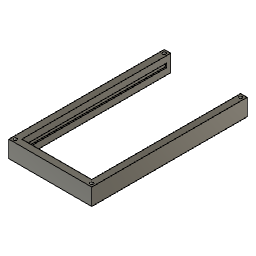
STM Holder v1 (Autodesk Fusion 360 design; units mm, degrees)
Autodesk Fusion 360 part; units mm, degrees
sketch "Sketch1" plane through (0, 0, 0) normal (0, 0, 1) x (1, 0, 0)
  line L0 (16.12, 50) -> (16.12, -69.76)
  line L1 (16.12, -69.76) -> (80, -69.76)
  line L2 (80, -69.76) -> (80, 50)
  line L3 (80, 50) -> (75, 50)
  line L4 (75, 50) -> (75, -64.76)
  line L5 (75, -64.76) -> (21.12, -64.76)
  line L6 (21.12, -64.76) -> (21.12, 50)
  line L7 (21.12, 50) -> (16.12, 50)
  circle A0 centre (18.62, 47.5) radius 1.25
  circle A1 centre (77.5, 47.5) radius 1.25
  circle A2 centre (18.62, -67.26) radius 1.25
  circle A3 centre (77.5, -67.26) radius 1.25
  dimension "d9" = 5
  dimension "d10" = 5
  dimension "d11" = 5
  dimension "d12" = 119.76
  dimension "d13" = 63.88
  dimension "d16" = 2.5
  dimension "d17" = 2.5
  dimension "d18" = 2.5
  dimension "d19" = 2.5
  dimension "d20" = 2.5
  dimension "d21" = 2.5
  dimension "d22" = 2.5
  dimension "d23" = 2.5
  dimension "d24" = 2.5
  dimension "d25" = 2.5
  dimension "d26" = 2.5
  dimension "d27" = 2.5
  dimension "d39" = 114.76
  constraint vertical L0
  constraint perpendicular L0 L1
  constraint perpendicular L1 L2
  constraint perpendicular L2 L3
  constraint perpendicular L3 L4
  constraint perpendicular L4 L5
  constraint perpendicular L5 L6
  constraint perpendicular L0 L7
  measures "d9" distance of L0.start L6.end
  measures "d10" distance of L2.end L3.end
  measures "d11" distance of L1 L4.end
  measures "d12" distance of L0.start L0.end
  measures "d13" distance of L0.end L1.end
  measures "d16" diameter of A0
  measures "d17" diameter of A1
  measures "d18" diameter of A2
  measures "d19" diameter of A3
  measures "d20" distance of L1 A2.centre
  measures "d21" distance of L0 A2.centre
  measures "d22" distance of L2 A3.centre
  measures "d23" distance of L1 A3.centre
  measures "d24" distance of L3 A1.centre
  measures "d25" distance of L2 A1.centre
  measures "d26" distance of L7 A0.centre
  measures "d27" distance of L0 A0.centre
  measures "d39" distance of L3.end L4.end
extrude "Extrude2" add sketch "Sketch1" along normal blind 18
sketch "Sketch3" plane through (0, 50, 0) normal (0, 1, 0) x (-1, 0, 0)
  line L0 (-80, 0) -> (-75, 0)
  line L1 (-75, 0) -> (-75, 18)
  line L2 (-75, 18) -> (-80, 18)
  line L3 (-80, 18) -> (-80, 0)
  line L4 (-75, 10) -> (-76, 10)
  line L5 (-76, 10) -> (-76, 13)
  line L6 (-76, 13) -> (-75, 13)
  line L7 (-75, 13) -> (-75, 10)
  dimension "d34" = 3
  dimension "d35" = 1
  dimension "d36" = 5
  constraint horizontal L4
  constraint vertical L5
  constraint horizontal L6
  constraint vertical L7
  constraint coincident L1 L4.start
  measures "d34" distance of L4.start L6.end
  measures "d35" distance of L4.start L4.end
  measures "d36" distance of L1.end L6.end
extrude "Extrude3" cut sketch "Sketch3" against normal blind 115.76 contours L1 L4 L5 L6 L7
sketch "Sketch4" plane through (0, -64.76, 0) normal (0, 1, 0) x (-1, 0, 0)
  line L0 (-75, 0) -> (-21.12, 0)
  line L1 (-21.12, 0) -> (-21.12, 18)
  line L2 (-21.12, 18) -> (-75, 18)
  line L3 (-75, 18) -> (-75, 13)
  line L4 (-75, 13) -> (-75, 10)
  line L5 (-75, 10) -> (-75, 0)
  line L6 (-75, 13) -> (-21.12, 13)
  line L7 (-21.12, 13) -> (-21.12, 9)
  line L8 (-21.12, 9) -> (-75, 9)
  line L9 (-75, 9) -> (-75, 13)
  constraint horizontal L6
  constraint vertical L7
  constraint horizontal L8
  constraint vertical L9
  constraint midpoint L1 L7.end
  constraint coincident L3.end L4.start
extrude "Extrude4" cut sketch "Sketch4" against normal blind 1 contours L1 L4 L5 L6 L7 L8 L9
sketch "Sketch5" plane through (0, 50, 0) normal (0, 1, 0) x (-1, 0, 0)
  line L0 (-21.12, 0) -> (-16.12, 0)
  line L1 (-16.12, 0) -> (-16.12, 18)
  line L2 (-16.12, 18) -> (-21.12, 18)
  line L3 (-21.12, 18) -> (-21.12, 0)
  line L4 (-21.12, 13) -> (-20.12, 13)
  line L5 (-20.12, 13) -> (-20.12, 10)
  line L6 (-20.12, 10) -> (-21.12, 10)
  line L7 (-21.12, 10) -> (-21.12, 13)
  dimension "d42" = 3
  dimension "d43" = 5
  dimension "d44" = 1
  constraint horizontal L4
  constraint vertical L5
  constraint horizontal L6
  constraint vertical L7
  constraint coincident L3 L4.start
  measures "d42" distance of L4.start L6.end
  measures "d43" distance of L2 L4
  measures "d44" distance of L5.end L6.end
extrude "Extrude5" cut sketch "Sketch5" against normal blind 115.76 contours L3 L4 L5 L6 L7
sketch "Sketch6" plane through (0, 0, 10) normal (0, 0, 1) x (-1, 0, 0)
  line L0 (-21.12, 65.76) -> (-21.12, -50)
  line L1 (-21.12, -50) -> (-20.12, -50)
  line L2 (-20.12, -50) -> (-20.12, 65.76)
  line L3 (-20.12, 65.76) -> (-21.12, 65.76)
  line L4 (-20.12, -50) -> (-21.12, -50)
  line L5 (-21.12, -50) -> (-21.12, -46)
  line L6 (-21.12, -46) -> (-20.12, -46)
  line L7 (-20.12, -46) -> (-20.12, -50)
  dimension "d47" = 4
  constraint horizontal L4
  constraint vertical L5
  constraint horizontal L6
  constraint vertical L7
  constraint coincident L1.end L2.start
  measures "d47" distance of L1.end L6.end
extrude "Extrude6" add sketch "Sketch6" along normal blind 2 contours L0 L1 L2 L4 L5 L6 L7
sketch "Sketch7" plane through (0, 0, 10) normal (0, 0, 1) x (-1, 0, 0)
  line L0 (-20.12, 65.76) -> (-21.12, 65.76)
  line L1 (-75, -50) -> (-76, -50)
  line L2 (-76, -50) -> (-76, -46)
  line L3 (-76, -46) -> (-75, -46)
  line L4 (-75, -46) -> (-75, -50)
  line L5 (-21.12, -46) -> (-20.12, -46)
  line L6 (-20.12, -46) -> (-20.12, 65.76)
  line L7 (-21.12, 65.76) -> (-21.12, -46)
  constraint horizontal L1
  constraint vertical L2
  constraint horizontal L3
  constraint vertical L4
extrude "Extrude9" add 1 faces at (39.08, -65.0933, 9) along direction (0, 0, 1) blind 1
extrude "Extrude10" add 1 faces at (20.7867, 47.3333, 12) along direction (0, 0, 1) blind 1
extrude "Extrude11" add sketch "Sketch7" along normal blind 3 contours L1 L2 L3 L4
extrude "Extrude12" cut 1 faces at (20.4533, 46, 12) along direction (0, 1, 0) blind 1
extrude "Extrude13" cut 1 faces at (75.6667, 46, 11) along direction (0, 1, 0) blind 1
extrude "Extrude14" cut 1 faces at (77.057, -28.1733, 0) along direction (0, 0, 1) blind 5
extrude "Extrude7" [suppressed]
extrude "Extrude8" [suppressed]
